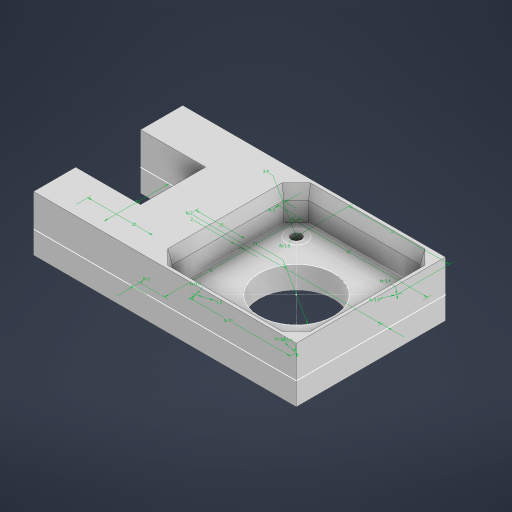
# Autodesk Inventor part: Z Stepper Holder
Saved by Autodesk Inventor 2024.2 (Build 282272000, 272)
## iProperties
Created: 2024-10-05
Part Number: Z Stepper Holder
Material: Generic
Document SubType Name: Modeling
Designer: jerem
Density: 1 g/cm^3
Appearance: Default
Author: jerem
Autodesk Inventor part; units mm, degrees
ref_plane "YZ Plane" through (0, 0, 0) normal (1, 0, 0) x (0, 1, 0)
ref_plane "XZ Plane" through (0, 0, 0) normal (0, 1, 0) x (-1, 0, 0)
ref_plane "XY Plane" through (0, 0, 0) normal (0, 0, 1) x (1, 0, 0)
sketch "Sketch1" plane through (0, 0, 0) normal (0, 1, 0) x (-1, 0, 0)
  line L0 (-21, 21) -> (21, 21)
  line L1 (21, 21) -> (21, -21)
  line L2 (21, -21) -> (-21, -21)
  line L3 (-21, -21) -> (-21, 21)
  line L4 (-21, 21) -> (21, -21) construction
  line L5 (21, 21) -> (-21, -21) construction
  circle A0 centre (15.5, -15.5) radius 1.7
  circle A1 centre (-15.5, -15.5) radius 1.7
  line L6 (15.5, -15.5) -> (-15.5, -15.5) construction
  circle A2 centre (15.5, 15.5) radius 1.7
  line L7 (15.5, 15.5) -> (-15.5, 15.5) construction
  circle A3 centre (-15.5, 15.5) radius 1.7
  line L8 (-23, 23) -> (23, 23)
  line L9 (23, 23) -> (23, -23)
  line L10 (23, -23) -> (-23, -23)
  line L11 (-23, -23) -> (-23, 23)
  circle A4 centre (0, 0) radius 11.5
  line L12 (23, 23) -> (-23, 23)
  circle A5 centre (15.5, 15.5) radius 3.2
  circle A6 centre (-15.5, 15.5) radius 3.2
  circle A7 centre (-15.5, -15.5) radius 3.2
  circle A8 centre (15.5, -15.5) radius 3.2
  line L13 (23, 23) -> (58, 23)
  line L14 (58, 23) -> (58, 10)
  line L15 (58, 10) -> (23, 10)
  line L16 (23, 10) -> (23, 23)
  line L17 (23, -23) -> (58, -23)
  line L18 (58, -23) -> (58, -10)
  line L19 (58, -10) -> (23, -10)
  line L20 (23, -10) -> (23, -23)
  line L21 (38, -10) -> (38, 10)
  dimension "d20" = 31
  dimension "d21" = 42
  dimension "d22" = 42
  dimension "d23" = 3.4
  dimension "d24" = 3.4
  dimension "d25" = 3.4
  dimension "d26" = 31
  dimension "d27" = 3.4
  dimension "d28" = 2
  dimension "d29" = 2
  dimension "d30" = 2
  dimension "d31" = 2
  dimension "d32" = 23
  dimension "d60" = 1.5
  dimension "d61" = 1.5
  dimension "d62" = 1.5
  dimension "d63" = 1.5
  dimension "d74" = 15
  dimension "d75" = 20
  dimension "d76" = 20
  constraints: 44 end point, 9 centre point, 8 parallel, 7 horizontal, 7 point on line, 5 perpendicular, 2 coincident, 2 midpoint, 1 collinear
  measures "d20" distance of L6.end L6.start
  measures "d21" distance of L1.end L2.end
  measures "d22" distance of L0.end L1.end
  measures "d23" diameter of A0
  measures "d24" diameter of A1
  measures "d25" diameter of A2
  measures "d26" distance of L7.start L7.end
  measures "d27" diameter of A3
  measures "d28" distance between parallel lines of L9 L1
  measures "d29" distance between parallel lines of L8 L0
  measures "d30" distance between parallel lines of L10 L2
  measures "d31" distance between parallel lines of L11 L3
  measures "d32" diameter of A4
  measures "d60" radial gap between concentric circles of A2 A5
  measures "d61" radial gap between concentric circles of A6 A3
  measures "d62" radial gap between concentric circles of A1 A7
  measures "d63" radial gap between concentric circles of A0 A8
  measures "d74" distance between parallel lines of L9 L21
  measures "d75" distance between parallel lines of L21 L14
  measures "d76" distance between parallel lines of L15 L19
extrude "Extrusion1" add sketch "Sketch1" along normal blind 10 contours L8 L9 L10 L11 | L13 L14 L15 L9 | L15 L21 L19 L9 | L9 L19 L18 L17
extrude "Extrusion2" add sketch "Sketch1" against normal blind 7 contours L0 L1 L2 L3 | L8 L9 L10 L11 | L13 L14 L15 L9 | L15 L21 L19 L9 | L9 L19 L18 L17 | A5 | A6 | A7 | A8
chamfer "Chamfer1" distance 3.8 angle 45 4 edges at (-21, 5, 21) (-21, 5, -21) (21, 5, -21) (21, 5, 21)
chamfer "Chamfer2" distance 1 distance2 4 8 edges at (0, 10, -21) (19.1, 10, -19.1) (21, 10, 0) (19.1, 10, 19.1) (0, 10, 21) (-21, 10, 0) (-19.1, 10, -19.1) (-19.1, 10, 19.1) measured on face at (-26.6667, 10, 3.3333)
extrude "Extrusion3" cut sketch "Sketch1" along normal blind 2 from surface at -7 contours A3 | A5 | A6 | A7 | A8
equation "\"d24\" = d23"
equation "\"d25\" = d23"
equation "\"d26\" = d20"
equation "\"d27\" = d23"
equation "\"d29\" = d28"
equation "\"d30\" = d31"
body "Solid1"
